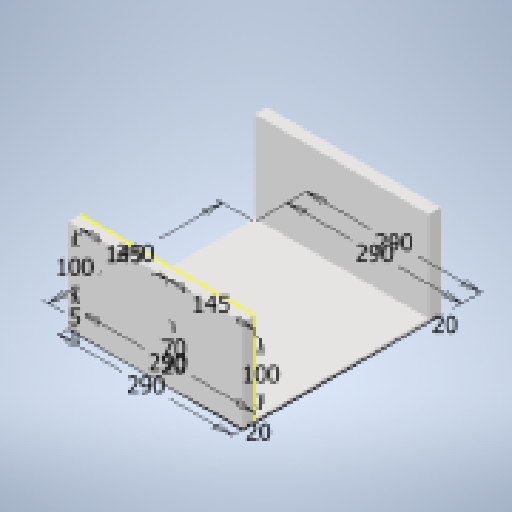
# Autodesk Inventor part: maze_test_course
Saved by Autodesk Inventor 2025 (Build 290162000, 162)
## iProperties
Created: 2026-06-30
Part Number: maze_test_course
Material: Типовые
Document SubType Name: Modeling
Designer: garin
Density: 1 g/cm^3
Appearance: По умолчанию
Author: garin
Autodesk Inventor part; units mm, degrees
ref_plane "YZ Plane" through (0, 0, 0) normal (1, 0, 0) x (0, 1, 0)
ref_plane "XZ Plane" through (0, 0, 0) normal (0, 1, 0) x (-1, 0, 0)
ref_plane "XY Plane" through (0, 0, 0) normal (0, 0, 1) x (1, 0, 0)
sketch "Эскиз1" plane through (0, 0, 0) normal (0, 1, 0) x (-1, 0, 0)
  line L0 (-145, 145) -> (145, 145)
  line L1 (145, 145) -> (145, -145)
  line L2 (145, -145) -> (-145, -145)
  line L3 (-145, -145) -> (-145, 145)
  line L4 (145, 0) -> (-145, 0) construction
  line L5 (0, 145) -> (0, -145) construction
  line L6 (145, 145) -> (-145, 145)
  line L7 (-145, 145) -> (-145, 165)
  line L8 (-145, 165) -> (145, 165)
  line L9 (145, 165) -> (145, 145)
  line L10 (145, -145) -> (-145, -145)
  line L11 (-145, -145) -> (-145, -165)
  line L12 (-145, -165) -> (145, -165)
  line L13 (145, -165) -> (145, -145)
  point P0 (0, 0)
  point P1 (0, 0)
  dimension "d0" = 290
  dimension "d1" = 290
  dimension "d2" = 290
  dimension "d3" = 20
  dimension "d4" = 290
  dimension "d5" = 20
  constraints: 28 end point, 6 parallel, 5 midpoint, 3 horizontal, 3 perpendicular, 1 coincident
  measures "d0" distance of L1.end L2.end
  measures "d1" distance of L0.end L1.end
  measures "d2" distance of L7.end L8.end
  measures "d3" distance of L6.end L7.end
  measures "d4" distance of L12.end L11.end
  measures "d5" distance of L11.end L10.end
extrude "Выдавливание1" add sketch "Эскиз1" along normal blind 5 contours L0 L1 L2 L3
extrude "Выдавливание2" add sketch "Эскиз1" along normal blind 155 contours L7 L8 L9 L0 | L2 L13 L12 L11
sketch "Эскиз2" plane through (145, 5, 145) normal (0, 0, -1) x (-1, 0, 0)
  line L0 (0, -5) -> (0, 150) projected
  line L1 (0, -5) -> (290, -5)
  line L2 (290, -5) -> (290, 0)
  line L3 (290, 0) -> (0, 0)
  line L4 (0, 0) -> (0, -5)
  line L5 (145, 0) -> (145, 150) construction
  line L6 (290, 150) -> (0, 150) projected
  line L7 (145, 0) -> (145, 70) construction
  line L8 (145, 0) -> (145, 20) construction
  line L9 (145, 20) -> (0, 20)
  line L10 (0, 20) -> (0, 120)
  line L11 (0, 120) -> (145, 120)
  line L12 (145, 120) -> (145, 20)
  line L13 (145, 20) -> (290, 20)
  line L14 (290, 20) -> (290, 120)
  line L15 (290, 120) -> (145, 120)
  line L16 (145, 120) -> (145, 20)
  point P0 (145, -5)
  dimension "d10" = 290
  dimension "d11" = 5
  dimension "d12" = 70
  dimension "d13" = 20
  dimension "d14" = 145
  dimension "d15" = 100
  dimension "d16" = 145
  dimension "d17" = 100
  constraints: 30 end point, 6 parallel, 3 horizontal, 3 perpendicular, 2 midpoint, 2 point on line
  measures "d10" distance of L3.end L2.end
  measures "d11" distance of L2.end L1.end
  measures "d12" distance of L5.start L7.end
  measures "d13" distance of L5.start L8.end
  measures "d14" distance of L10.end L11.end
  measures "d15" distance of L9.end L10.end
  measures "d16" distance of L15.end L14.end
  measures "d17" distance of L14.end L13.end
